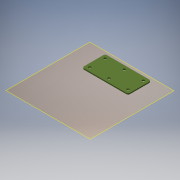
# Autodesk Inventor part: Board
Saved by Autodesk Inventor 2016 (Build 200138000, 138)
## iProperties
Created: 2015-07-14
Part Number: Board
Material: Generic
Document SubType Name: Modeling
Designer: 3DPrinterUser
Density: 1 g/cm^3
Appearance: Olive Green
Author: 3DPrinterUser
Autodesk Inventor part; units mm, degrees
ref_plane "YZ Plane" through (0, 0, 0) normal (1, 0, 0) x (0, 1, 0)
ref_plane "XZ Plane" through (0, 0, 0) normal (0, 1, 0) x (-1, 0, 0)
ref_plane "XY Plane" through (0, 0, 0) normal (0, 0, 1) x (1, 0, 0)
ref_plane "Work Plane1" through (0, 0, 6) normal (0, 0, 1) x (1, 0, 0)
sketch "Sketch2" plane through (0, 0, 6) normal (0, 0, 1) x (1, 0, 0)
  circle A0 centre (30, 51.3034) radius 1.5 construction
  circle A1 centre (30, 27.3034) radius 1.5 construction
  circle A2 centre (0, 51.3034) radius 1.5 construction
  circle A3 centre (0, 27.3034) radius 1.5 construction
  circle A4 centre (-30, 51.3034) radius 1.5 construction
  circle A5 centre (-30, 27.3034) radius 1.5 construction
  line L0 (36, 57.3034) -> (-36, 57.3034)
  line L1 (-36, 57.3034) -> (-36, 21.3034)
  line L2 (-36, 21.3034) -> (36, 21.3034)
  line L3 (36, 21.3034) -> (36, 57.3034)
  circle A6 centre (30, 51.3034) radius 1.9
  circle A7 centre (30, 27.3034) radius 1.9
  circle A8 centre (0, 51.3034) radius 1.9
  circle A9 centre (0, 27.3034) radius 1.9
  circle A10 centre (-30, 51.3034) radius 1.9
  circle A11 centre (-30, 27.3034) radius 1.9
  point P0 (0, 0)
  dimension "d0" = 6
  dimension "d1" = 6
  dimension "d2" = 6
  dimension "d3" = 6
  dimension "d4" = 0.4
  dimension "d5" = 0.4
  dimension "d6" = 0.4
  dimension "d7" = 0.4
  dimension "d8" = 0.4
  dimension "d9" = 0.4
  constraints: 8 end point, 6 centre point, 2 parallel, 1 horizontal, 1 perpendicular
  measures "d0" distance from line of L0 A0.centre
  measures "d1" distance from line of L3 A0.centre
  measures "d2" distance from line of L1 A5.centre
  measures "d3" distance from line of L2 A5.centre
  measures "d4" radial gap between concentric circles of A0 A6
  measures "d5" radial gap between concentric circles of A1 A7
  measures "d6" radial gap between concentric circles of A2 A8
  measures "d7" radial gap between concentric circles of A3 A9
  measures "d8" radial gap between concentric circles of A4 A10
  measures "d9" radial gap between concentric circles of A5 A11
extrude "Extrusion1" add sketch "Sketch2" along normal blind 1.75
fillet "Fillet1" radius 3 4 edges at (-36, 57.3034, 6.875) (-36, 21.3034, 6.875) (36, 57.3034, 6.875) (36, 21.3034, 6.875)
body "Solid1"
